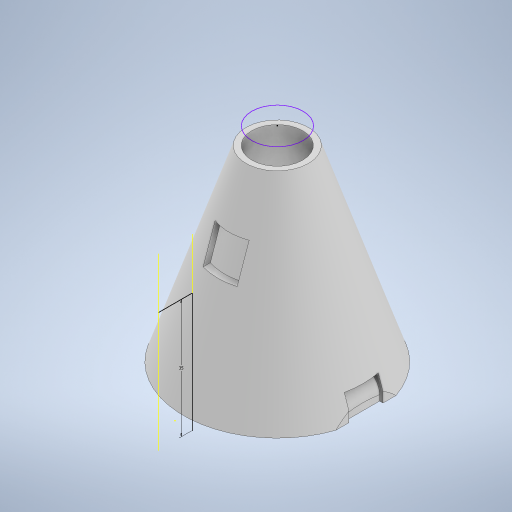
# Autodesk Inventor part: cone_p3_testpart1
Saved by Autodesk Inventor 2024 (Build 280153000, 153)
## iProperties
Created: 2023-09-28
Part Number: cone_p3_testpart1
Material: Generic
Document SubType Name: Modeling
Designer: kubad
Density: 1 g/cm^3
Appearance: Default
Author: kubad
## iProperties of the stored document cone_p3_testpart1_3DPrint.ipt
Created: 2023-09-28
Part Number: cone_p3_testpart1_3DPrint
Material: Generic
Document SubType Name: Modeling
Designer: kubad
Density: 1 g/cm^3
Appearance: Default
Author: kubad
Autodesk Inventor part; units mm, degrees
ref_plane "YZ Plane" through (0, 0, 0) normal (1, 0, 0) x (0, 1, 0)
ref_plane "XZ Plane" through (0, 0, 0) normal (0, 1, 0) x (-1, 0, 0)
ref_plane "XY Plane" through (0, 0, 0) normal (0, 0, 1) x (1, 0, 0)
sketch "Sketch1" plane through (0, 0, 0) normal (0, 1, 0) x (-1, 0, 0)
  point P0 (0, 0)
sketch "Sketch2" plane through (0, 0, 0) normal (0, 1, 0) x (-1, 0, 0)
  circle A0 centre (0, 0) radius 7.5
  dimension "d0" = 15
  constraints: 1 centre point, 1 coincident
  measures "d0" diameter of A0
extrude "Extrusion1" add sketch "Sketch2" along normal blind 60
sketch "Sketch3" plane through (0, 60, 0) normal (0, 1, 0) x (1, 0, 0)
  circle A0 centre (0, 0) radius 7.5
  constraints: 1 centre point, 1 coincident
sketch "Sketch4" plane through (0, 0, 0) normal (0, -1, 0) x (1, 0, 0)
  circle A0 centre (0, 0) radius 25
  circle A1 centre (0, 0) radius 7.5 projected
  circle A2 centre (0, 0) radius 27.5
  dimension "d3" = 50
  dimension "d4" = 55
  constraints: 2 centre point, 2 coincident
  measures "d3" diameter of A0
  measures "d4" diameter of A2
loft "Loft1" add profiles "Sketch4" section 1 edges at (7.5, 60, 0) contours A0 | A1 | A2
sketch "Sketch5" plane through (0, 0, 0) normal (0, -1, 0) x (1, 0, 0)
  circle A0 centre (0, 0) radius 7.5 projected
  circle A1 centre (0, 0) radius 27.5
  circle A2 centre (0, 0) radius 25
  circle A3 centre (0, 0) radius 7.5
  dimension "d9" = 50
  dimension "d10" = 15
  constraints: 3 centre point, 3 coincident
  measures "d9" diameter of A2
  measures "d10" diameter of A3
sketch "Sketch6" plane through (0, 60, 0) normal (0, 1, 0) x (1, 0, 0)
  circle A0 centre (0, 0) radius 7.5
  constraints: 1 centre point, 1 coincident
extrude "Extrusion2" cut sketch "Sketch6" against normal blind 5
sketch "Sketch7" plane through (0, 55, 0) normal (0, 1, 0) x (1, 0, 0)
  circle A0 centre (0, 0) radius 7.5
  line L0 (-11.197, -10.4421) -> (10.2744, -10.4421)
  line L1 (10.2744, -10.4421) -> (10.2744, 11.5325)
  line L2 (10.2744, 11.5325) -> (-11.197, 11.5325)
  line L3 (-11.197, 11.5325) -> (-11.197, -10.4421)
  constraints: 8 end point, 2 parallel, 1 centre point, 1 coincident, 1 horizontal, 1 perpendicular
loft "Loft2" cut profiles "Sketch5" section 1 edges at (-7.5, 55, 0) contours A0 | A2
extrude "Extrusion3" cut sketch "Sketch7" along normal through all
sketch "Sketch8" plane through (0, 0, 0) normal (0, -1, 0) x (1, 0, 0)
  circle A0 centre (0, 0) radius 25
  circle A1 centre (0, 0) radius 27.5
  line L0 (27.5, 0) -> (27.5, -5)
  line L1 (27.0416, -5) -> (26.0416, -5)
  line L2 (26.0416, -5) -> (26.0416, 5)
  line L3 (26.0416, 5) -> (27.0416, 5)
  line L4 (27.0416, 5) -> (27.0416, -5)
  line L5 (-27.5, 0) -> (-27.5, -5)
  line L6 (-27.0416, -5) -> (-26.0416, -5)
  line L7 (-26.0416, -5) -> (-26.0416, 5)
  line L8 (-26.0416, 5) -> (-27.0416, 5)
  line L9 (-27.0416, 5) -> (-27.0416, -5)
  line L10 (26.0416, -5) -> (25.0416, -5)
  line L11 (25.0416, -5) -> (25.0416, 5)
  line L12 (25.0416, 5) -> (26.0416, 5)
  line L13 (26.0416, 5) -> (26.0416, -5)
  line L14 (-26.0416, -5) -> (-25.0416, -5)
  line L15 (-25.0416, -5) -> (-25.0416, 5)
  line L16 (-25.0416, 5) -> (-26.0416, 5)
  line L17 (-26.0416, 5) -> (-26.0416, -5)
  line L18 (-26.0416, 5) -> (-26.0416, 8.8365)
  line L19 (-26.0416, -5) -> (-26.0416, -8.8365)
  line L20 (26.0416, -5) -> (26.0416, -8.8365)
  line L21 (26.0416, 5) -> (26.0416, 8.8365)
  circle A2 centre (0, 0) radius 27.5 projected
  dimension "d19" = 5
  dimension "d20" = 1
  dimension "d21" = 10
  dimension "d22" = 5
  dimension "d23" = 1
  dimension "d24" = 10
  dimension "d25" = 1
  dimension "d26" = 1
  constraints: 44 end point, 9 parallel, 4 horizontal, 4 perpendicular, 3 vertical, 2 coincident, 2 point on line, 1 centre point, 11 other
  measures "d19" distance of L0.start L0.end
  measures "d20" distance of L2.end L3.end
  measures "d21" distance of L1.end L2.end
  measures "d22" distance of L5.start L5.end
  measures "d23" distance of L8.end L7.end
  measures "d24" distance of L7.end L6.end
  measures "d25" distance of L11.end L12.end
  measures "d26" distance of L16.end L15.end
extrude "Extrusion4" cut sketch "Sketch8" against normal through all contours A1 L4 | L3 L21 A1 | L4 L1 L2 L3 | A1 L20 L1 | L18 L8 A1 | A1 L6 L19 | L9 A1 | L8 L7 L6 L9
sketch "Sketch9" plane through (0, 0, 0) normal (0, -1, 0) x (1, 0, 0)
  circle A0 centre (0, 0) radius 27.5
  circle A1 centre (0, 0) radius 25
  line L0 (27.5, 0) -> (27.5, -5)
  line L1 (26.0416, -8.8365) -> (26.0416, 8.8365) projected
  line L2 (27.0416, -5) -> (26.0416, -5)
  line L3 (26.0416, -5) -> (26.0416, 5)
  line L4 (26.0416, 5) -> (27.0416, 5)
  line L5 (27.0416, 5) -> (27.0416, -5)
  line L6 (26.0416, 5) -> (25.0416, 5)
  line L7 (25.0416, 5) -> (25.0416, -5)
  line L8 (25.0416, -5) -> (26.0416, -5)
  line L9 (26.0416, -5) -> (26.0416, 5)
  line L10 (-27.5, 0) -> (-27.5, -5)
  line L11 (-26.0416, 8.8365) -> (-26.0416, -8.8365) projected
  line L12 (-27.0416, -5) -> (-26.0416, -5)
  line L13 (-26.0416, -5) -> (-26.0416, 5)
  line L14 (-26.0416, 5) -> (-27.0416, 5)
  line L15 (-27.0416, 5) -> (-27.0416, -5)
  line L16 (-26.0416, -5) -> (-25.0416, -5)
  line L17 (-25.0416, -5) -> (-25.0416, 5)
  line L18 (-25.0416, 5) -> (-26.0416, 5)
  line L19 (-26.0416, 5) -> (-26.0416, -5)
  dimension "d29" = 5
  dimension "d30" = 10
  dimension "d31" = 1
  dimension "d32" = 5
  dimension "d33" = 10
  dimension "d34" = 1
  constraints: 36 end point, 8 parallel, 4 horizontal, 4 perpendicular, 3 point on line, 3 vertical, 2 coincident, 1 centre point, 6 other
  measures "d29" distance of L0.start L0.end
  measures "d30" distance of L2.end L3.end
  measures "d31" distance of L8.end L7.end
  measures "d32" distance of L10.start L10.end
  measures "d33" distance of L13.end L12.end
  measures "d34" distance of L18.end L17.end
extrude "Extrusion5" cut sketch "Sketch9" against normal blind 7 contours L1 L8 L7 L6 | L18 L17 L16 L11
sketch "Sketch10" plane through (25.0416, 0, 5) normal (1, 0, 0) x (0, 0, -1)
  line L0 (0, 0) -> (10, 0)
  line L1 (10, 0) -> (10, 7)
  line L2 (10, 7) -> (0, 7)
  line L3 (0, 7) -> (0, 0)
  line L4 (10, 7) -> (0, 7)
  line L5 (0, 7) -> (0, 6)
  line L6 (0, 6) -> (10, 6)
  line L7 (10, 6) -> (10, 7)
  point P0 (5, 0)
  dimension "d37" = 10
  dimension "d38" = 7
  dimension "d39" = 1
  constraints: 16 end point, 4 parallel, 2 horizontal, 2 perpendicular, 1 point on line
  measures "d37" distance of L2.end L1.end
  measures "d38" distance of L1.end L0.end
  measures "d39" distance of L5.end L4.end
extrude "Extrusion6" cut sketch "Sketch10" against normal through all contours L3 L2 L1 L6
fillet "Fillet1" radius 5 1 edges at (25.0416, 6, 0)
fillet "Fillet2" radius 5 1 edges at (-25.0416, 6, 0)
sketch "Sketch11" plane through (0, 0, 0) normal (0, -1, 0) x (1, 0, 0)
  line L0 (0, 0) -> (35, 0)
  line L1 (35, 0) -> (-35, 0)
  line L2 (-35, 0) -> (-35, 30)
  line L3 (-35, 30) -> (35, 30)
  line L4 (35, 30) -> (35, 0)
  line L5 (0, 30) -> (5, 30)
  line L6 (5, 30) -> (-5, 30)
  line L7 (-5, 30) -> (-5, 40)
  line L8 (-5, 40) -> (5, 40)
  line L9 (5, 40) -> (5, 30)
  dimension "d44" = 35
  dimension "d45" = 70
  dimension "d46" = 30
  dimension "d47" = 5
  dimension "d48" = 10
  dimension "d49" = 10
  constraints: 20 end point, 4 parallel, 3 horizontal, 2 perpendicular, 1 midpoint, 1 point on line
  measures "d44" distance of L0.start L0.end
  measures "d45" distance of L2.end L3.end
  measures "d46" distance of L1.end L2.end
  measures "d47" distance of L5.start L5.end
  measures "d48" distance of L7.end L8.end
  measures "d49" distance of L6.end L7.end
extrude "Extrusion7" add sketch "Sketch11" against normal blind 50 contours L3 L7 L8 L9
sketch "Sketch12" plane through (5, 0, 40) normal (1, 0, 0) x (0, 0, -1)
  line L0 (10, 0) -> (10, 50) projected
  line L1 (10, 0) -> (10, 35)
  line L2 (10, 35) -> (0, 35)
  line L3 (0, 0) -> (0, 50) projected
  point P0 (40, 0)
  dimension "d52" = 35
  constraints: 4 end point, 2 point on line, 1 horizontal
  measures "d52" distance of L0.start L1.end
sketch "Sketch13" plane through (5, 0, 30) normal (0, 0, -1) x (-1, 0, 0)
  point P0 (5, 0)
sketch "Sketch14" plane through (-5, 0, 40) normal (0, 0, 1) x (1, 0, 0)
  line L0 (10, 0) -> (10, 50) projected
  line L1 (10, 35) -> (10, 40)
  line L2 (0, 0) -> (0, 50) projected
  line L3 (10, 40) -> (0, 40)
  line L4 (0, 40) -> (0, 30)
  line L5 (0, 30) -> (10, 30)
  line L6 (10, 30) -> (10, 40)
  point P0 (5, 0)
  dimension "d53" = 5
  dimension "d54" = 10
  constraints: 10 end point, 3 point on line, 2 parallel, 1 horizontal, 1 perpendicular
  measures "d53" distance of L1.start L1.end
  measures "d54" distance of L4.end L3.end
extrude "Extrusion8" cut sketch "Sketch14" against normal blind 35
sketch "Sketch15" plane through (0, 50, 0) normal (0, 1, 0) x (1, 0, 0)
  line L0 (5, -30) -> (-5, -30) projected
  line L1 (-5, -40) -> (5, -40) projected
  line L2 (-5, -30) -> (5, -30)
  line L3 (5, -30) -> (5, -40)
  line L4 (5, -40) -> (-5, -40)
  line L5 (-5, -40) -> (-5, -30)
  point P0 (0, 0)
  constraints: 8 end point, 2 parallel, 1 horizontal, 1 perpendicular
extrude "Extrusion9" cut sketch "Sketch15" against normal through all
body "Solid1"
